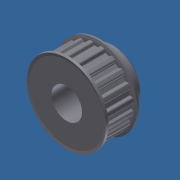
# Autodesk Inventor part: Synchrone Riemenscheibe2
Saved by Autodesk Inventor 2016 (Build 200138000, 138)
## iProperties
Created: 2015-01-06
Part Number: Synchrone Riemenscheibe2
Material: Steel
Document SubType Name: Modeling
Designer: 4ndreas
Density: 1 g/cm^3
Appearance: Steel
CustomPartVersion: 1
Author: 4ndreas
Autodesk Inventor part; units mm, degrees
ref_plane "YZ Plane" through (0, 0, 0) normal (1, 0, 0) x (0, 1, 0)
ref_plane "XZ Plane" through (0, 0, 0) normal (0, 1, 0) x (-1, 0, 0)
ref_plane "XY Plane" through (0, 0, 0) normal (0, 0, 1) x (1, 0, 0)
sketch "Riemenscheibenskizze" plane through (0, 0, 0) normal (0, 0, 1) x (1, 0, 0)
  circle A0 centre (0, 0) radius 15.9155 construction
  circle A1 centre (0, 0) radius 15.4155
  circle A2 centre (0, 0) radius 14.1655
  line L0 (-1.451, 15.3471) -> (-0.9, 14.1655)
  line L1 (-0.9, 14.1655) -> (0.9, 14.1655)
  line L2 (0.9, 14.1655) -> (1.451, 15.3471)
  line L3 (0, 0) -> (0, 15.4155) construction
  point P0 (0, 14.1655)
  dimension "d0" = 31.831
  dimension "d1" = 0.5
  dimension "d2" = 1.25
  dimension "d3" = 50
  dimension "d4" = 1.8
  constraints: 8 end point, 3 coincident, 3 point on circle, 2 centre point, 1 horizontal, 1 midpoint, 1 point on line, 1 vertical, 1 vertical alignment, 3 other
  measures "d0" diameter of A0
  measures "d1" radial gap between concentric circles of A0 A1
  measures "d3" angle of L2 L0
  measures "d4" distance of L0.end L1.end
extrude "Grundkörper" add sketch "Riemenscheibenskizze" along normal mid plane 18 contours A2 | A1 L0 L1 L2 | L2 L1 L0 A1
extrude "Zahn" cut sketch "Riemenscheibenskizze" along normal through all both and the other way through all contours L2 L1 L0 A1 picked at (0, 14.9938)
fillet "Fillet" radius 0.4 2 edges at (0.9, 14.1655, 0) (-0.9, 14.1655, 0)
fillet "Fillet" radius 0.6 4 edges at (-1.451, 15.3471, 4.5) (-1.451, 15.3471, -4.5) (1.451, 15.3471, 4.5) (1.451, 15.3471, -4.5)
pattern_circular "Zähne" count 20 over 360 about axis through (0, 0, -10) along (0, 0, 1) of "Zahn", "Fillet"
pulley flange "Flansch links" diameter 30.831 height 1.2 thickness 1 bend angle 10 centre (0, 0, -9) toward (0, 0, -1)
pulley flange "Flansch rechts" diameter 30.831 height 1.2 thickness 1 bend angle 10 centre (0, 0, 9) toward (0, 0, 1)
sketch "Skizze2" plane through (0, 0, -10) normal (0, 0, -1) x (-1, 0, 0)
  circle A0 centre (0, 0) radius 15.4155
  circle A1 centre (0, 0) radius 11.5
  circle A2 centre (0, 0) radius 15.4155 projected
  dimension "d17" = 23
  constraints: 2 centre point, 1 coincident
  measures "d17" diameter of A1
extrude "Extrusion3" add sketch "Skizze2" along normal blind 6 contours A1
chamfer "Fase1" distance 0.5 angle 45 1 edges at (11.5, 0, -16)
sketch "Skizze3" plane through (0, 0, -16) normal (0, 0, -1) x (-1, 0, 0)
  circle A0 centre (0, 0) radius 11 projected
hole "Bohrung1" at (0, 0, -16) direction (0, 0, 1) diameter 12.7 end through all
equation "\"d1\" = da_a"
equation "\"d2\" = da_hg"
equation "\"d3\" = 2 * da_fi"
equation "\"d4\" = da_bw"
equation "\"d5\" = da_bf"
equation "\"d7\" = da_bf"
equation "\"d9\" = da_rb"
equation "\"d10\" = da_rt"
equation "\"da_pb\" = 5"
equation "\"da_fi\" = 25deg"
equation "\"da_hg\" = 1.25"
equation "\"da_bw\" = 1.8"
equation "\"da_rb\" = 0.4"
equation "\"da_rt\" = 0.6"
equation "\"da_a\" = 0.5"
equation "\"da_bf\" = 18"
equation "\"da_wf\" = 1"
equation "\"da_hf\" = 1.2"
body "Solid1"
